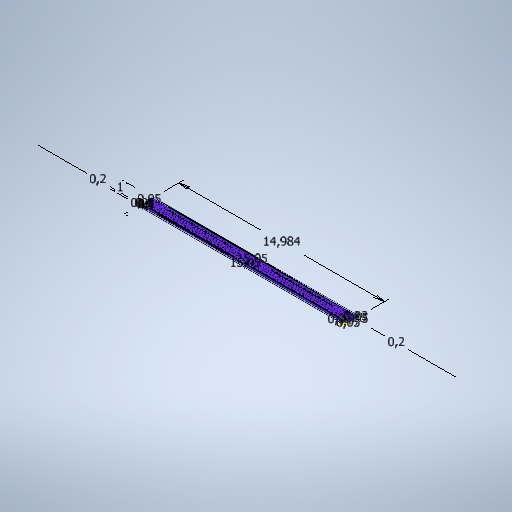
# Autodesk Inventor part: sensor_electrodo
Saved by Autodesk Inventor 2025.2 (Build 292293000, 293)
## iProperties
Created: 2025-03-24
Part Number: sensor_electrodo
Material: Genérico
Document SubType Name: Modeling
Designer: julia
Density: 1 g/cm^3
Appearance: Vidriado - Ladrillo refractario
Author: julia
Autodesk Inventor part; units mm, degrees
ref_plane "YZ Plane" through (0, 0, 0) normal (1, 0, 0) x (0, 1, 0)
ref_plane "XZ Plane" through (0, 0, 0) normal (0, 1, 0) x (-1, 0, 0)
ref_plane "XY Plane" through (0, 0, 0) normal (0, 0, 1) x (1, 0, 0)
sketch "Boceto1" plane through (0, 0, 0) normal (0, 1, 0) x (-1, 0, 0)
  line L0 (0, 0) -> (14.984, 0)
  line L1 (14.984, 0) -> (14.984, -1)
  line L2 (14.984, -1) -> (0, -1)
  line L3 (0, -1) -> (0, 0)
  line L4 (-0.05, -0.23) -> (0, -0.23)
  line L5 (-0.0448, -0.147) -> (-0.0448, -0.3192)
  line L6 (-0.0448, -0.23) -> (15.0052, -0.23)
  line L7 (15.0052, -0.23) -> (15.0052, -0.28)
  line L8 (15.0052, -0.28) -> (14.9052, -0.28)
  line L9 (14.9052, -0.28) -> (14.9052, -0.38)
  line L10 (14.9052, -0.38) -> (14.8052, -0.38)
  line L11 (14.8052, -0.38) -> (14.8052, -0.28)
  line L12 (14.8052, -0.28) -> (14.7052, -0.28)
  line L13 (14.7052, -0.28) -> (14.7052, -0.38)
  line L14 (14.7052, -0.38) -> (14.6052, -0.38)
  line L15 (14.6052, -0.38) -> (14.6052, -0.28)
  line L16 (14.6052, -0.28) -> (14.5052, -0.28)
  line L17 (14.5052, -0.28) -> (14.5052, -0.38)
  line L18 (14.5052, -0.38) -> (14.4052, -0.38)
  line L19 (14.4052, -0.38) -> (14.4052, -0.28)
  line L20 (14.4052, -0.28) -> (14.3052, -0.28)
  line L21 (14.3052, -0.28) -> (14.3052, -0.38)
  line L22 (14.3052, -0.38) -> (14.2052, -0.38)
  line L23 (14.2052, -0.38) -> (14.2052, -0.28)
  line L24 (14.2052, -0.28) -> (14.1052, -0.28)
  line L25 (14.1052, -0.28) -> (14.1052, -0.38)
  line L26 (14.1052, -0.38) -> (14.0052, -0.38)
  line L27 (14.0052, -0.38) -> (14.0052, -0.28)
  line L28 (14.0052, -0.28) -> (13.9052, -0.28)
  line L29 (13.9052, -0.28) -> (13.9052, -0.38)
  line L30 (13.9052, -0.38) -> (13.8052, -0.38)
  line L31 (13.8052, -0.38) -> (13.8052, -0.28)
  line L32 (13.8052, -0.28) -> (13.7052, -0.28)
  line L33 (13.7052, -0.28) -> (13.7052, -0.38)
  line L34 (13.7052, -0.38) -> (13.6052, -0.38)
  line L35 (13.6052, -0.38) -> (13.6052, -0.28)
  line L36 (13.6052, -0.28) -> (13.5052, -0.28)
  line L37 (13.5052, -0.28) -> (13.5052, -0.38)
  line L38 (13.5052, -0.38) -> (13.4052, -0.38)
  line L39 (13.4052, -0.38) -> (13.4052, -0.28)
  line L40 (13.4052, -0.28) -> (13.3052, -0.28)
  line L41 (13.3052, -0.28) -> (13.3052, -0.38)
  line L42 (13.3052, -0.38) -> (13.2052, -0.38)
  line L43 (13.2052, -0.38) -> (13.2052, -0.28)
  line L44 (13.2052, -0.28) -> (13.1052, -0.28)
  line L45 (13.1052, -0.28) -> (13.1052, -0.38)
  line L46 (13.1052, -0.38) -> (13.0052, -0.38)
  line L47 (13.0052, -0.38) -> (13.0052, -0.28)
  line L48 (13.0052, -0.28) -> (12.9052, -0.28)
  line L49 (12.9052, -0.28) -> (12.9052, -0.38)
  line L50 (12.9052, -0.38) -> (12.8052, -0.38)
  line L51 (12.8052, -0.38) -> (12.8052, -0.28)
  line L52 (12.8052, -0.28) -> (12.7052, -0.28)
  line L53 (12.7052, -0.28) -> (12.7052, -0.38)
  line L54 (12.7052, -0.38) -> (12.6052, -0.38)
  line L55 (12.6052, -0.38) -> (12.6052, -0.28)
  line L56 (12.6052, -0.28) -> (12.5052, -0.28)
  line L57 (12.5052, -0.28) -> (12.5052, -0.38)
  line L58 (12.5052, -0.38) -> (12.4052, -0.38)
  line L59 (12.4052, -0.38) -> (12.4052, -0.28)
  line L60 (12.4052, -0.28) -> (12.3052, -0.28)
  line L61 (12.3052, -0.28) -> (12.3052, -0.38)
  line L62 (12.3052, -0.38) -> (12.2052, -0.38)
  line L63 (12.2052, -0.38) -> (12.2052, -0.28)
  line L64 (12.2052, -0.28) -> (12.1052, -0.28)
  line L65 (12.1052, -0.28) -> (12.1052, -0.38)
  line L66 (12.1052, -0.38) -> (12.0052, -0.38)
  line L67 (12.0052, -0.38) -> (12.0052, -0.28)
  line L68 (12.0052, -0.28) -> (11.9052, -0.28)
  line L69 (11.9052, -0.28) -> (11.9052, -0.38)
  line L70 (11.9052, -0.38) -> (11.8052, -0.38)
  line L71 (11.8052, -0.38) -> (11.8052, -0.28)
  line L72 (11.8052, -0.28) -> (11.7052, -0.28)
  line L73 (11.7052, -0.28) -> (11.7052, -0.38)
  line L74 (11.7052, -0.38) -> (11.6052, -0.38)
  line L75 (11.6052, -0.38) -> (11.6052, -0.28)
  line L76 (11.6052, -0.28) -> (11.5052, -0.28)
  line L77 (11.5052, -0.28) -> (11.5052, -0.38)
  line L78 (11.5052, -0.38) -> (11.4052, -0.38)
  line L79 (11.4052, -0.38) -> (11.4052, -0.28)
  line L80 (11.4052, -0.28) -> (11.3052, -0.28)
  line L81 (11.3052, -0.28) -> (11.3052, -0.38)
  line L82 (11.3052, -0.38) -> (11.2052, -0.38)
  line L83 (11.2052, -0.38) -> (11.2052, -0.28)
  line L84 (11.2052, -0.28) -> (11.1052, -0.28)
  line L85 (11.1052, -0.28) -> (11.1052, -0.38)
  line L86 (11.1052, -0.38) -> (11.0052, -0.38)
  line L87 (11.0052, -0.38) -> (11.0052, -0.28)
  line L88 (11.0052, -0.28) -> (10.9052, -0.28)
  line L89 (10.9052, -0.28) -> (10.9052, -0.38)
  line L90 (10.9052, -0.38) -> (10.8052, -0.38)
  line L91 (10.8052, -0.38) -> (10.8052, -0.28)
  line L92 (10.8052, -0.28) -> (10.7052, -0.28)
  line L93 (10.7052, -0.28) -> (10.7052, -0.38)
  line L94 (10.7052, -0.38) -> (10.6052, -0.38)
  line L95 (10.6052, -0.38) -> (10.6052, -0.28)
  line L96 (10.6052, -0.28) -> (10.5052, -0.28)
  line L97 (10.5052, -0.28) -> (10.5052, -0.38)
  line L98 (10.5052, -0.38) -> (10.4052, -0.38)
  line L99 (10.4052, -0.38) -> (10.4052, -0.28)
  line L100 (10.4052, -0.28) -> (10.3052, -0.28)
  line L101 (10.3052, -0.28) -> (10.3052, -0.38)
  line L102 (10.3052, -0.38) -> (10.2052, -0.38)
  line L103 (10.2052, -0.38) -> (10.2052, -0.28)
  line L104 (10.2052, -0.28) -> (10.1052, -0.28)
  line L105 (10.1052, -0.28) -> (10.1052, -0.38)
  line L106 (10.1052, -0.38) -> (10.0052, -0.38)
  line L107 (10.0052, -0.38) -> (10.0052, -0.28)
  line L108 (10.0052, -0.28) -> (9.9052, -0.28)
  line L109 (9.9052, -0.28) -> (9.9052, -0.38)
  line L110 (9.9052, -0.38) -> (9.8052, -0.38)
  line L111 (9.8052, -0.38) -> (9.8052, -0.28)
  line L112 (9.8052, -0.28) -> (9.7052, -0.28)
  line L113 (9.7052, -0.28) -> (9.7052, -0.38)
  line L114 (9.7052, -0.38) -> (9.6052, -0.38)
  line L115 (9.6052, -0.38) -> (9.6052, -0.28)
  line L116 (9.6052, -0.28) -> (9.5052, -0.28)
  line L117 (9.5052, -0.28) -> (9.5052, -0.38)
  line L118 (9.5052, -0.38) -> (9.4052, -0.38)
  line L119 (9.4052, -0.38) -> (9.4052, -0.28)
  line L120 (9.4052, -0.28) -> (9.3052, -0.28)
  line L121 (9.3052, -0.28) -> (9.3052, -0.38)
  line L122 (9.3052, -0.38) -> (9.2052, -0.38)
  line L123 (9.2052, -0.38) -> (9.2052, -0.28)
  line L124 (9.2052, -0.28) -> (9.1052, -0.28)
  line L125 (9.1052, -0.28) -> (9.1052, -0.38)
  line L126 (9.1052, -0.38) -> (9.0052, -0.38)
  line L127 (9.0052, -0.38) -> (9.0052, -0.28)
  line L128 (9.0052, -0.28) -> (8.9052, -0.28)
  line L129 (8.9052, -0.28) -> (8.9052, -0.38)
  line L130 (8.9052, -0.38) -> (8.8052, -0.38)
  line L131 (8.8052, -0.38) -> (8.8052, -0.28)
  line L132 (8.8052, -0.28) -> (8.7052, -0.28)
  line L133 (8.7052, -0.28) -> (8.7052, -0.38)
  line L134 (8.7052, -0.38) -> (8.6052, -0.38)
  line L135 (8.6052, -0.38) -> (8.6052, -0.28)
  line L136 (8.6052, -0.28) -> (8.5052, -0.28)
  line L137 (8.5052, -0.28) -> (8.5052, -0.38)
  line L138 (8.5052, -0.38) -> (8.4052, -0.38)
  line L139 (8.4052, -0.38) -> (8.4052, -0.28)
  line L140 (8.4052, -0.28) -> (8.3052, -0.28)
  line L141 (8.3052, -0.28) -> (8.3052, -0.38)
  line L142 (8.3052, -0.38) -> (8.2052, -0.38)
  line L143 (8.2052, -0.38) -> (8.2052, -0.28)
  line L144 (8.2052, -0.28) -> (8.1052, -0.28)
  line L145 (8.1052, -0.28) -> (8.1052, -0.38)
  line L146 (8.1052, -0.38) -> (8.0052, -0.38)
  line L147 (8.0052, -0.38) -> (8.0052, -0.28)
  line L148 (8.0052, -0.28) -> (7.9052, -0.28)
  line L149 (7.9052, -0.28) -> (7.9052, -0.38)
  line L150 (7.9052, -0.38) -> (7.8052, -0.38)
  line L151 (7.8052, -0.38) -> (7.8052, -0.28)
  line L152 (7.8052, -0.28) -> (7.7052, -0.28)
  line L153 (7.7052, -0.28) -> (7.7052, -0.38)
  line L154 (7.7052, -0.38) -> (7.6052, -0.38)
  line L155 (7.6052, -0.38) -> (7.6052, -0.28)
  line L156 (7.6052, -0.28) -> (7.5052, -0.28)
  line L157 (7.5052, -0.28) -> (7.5052, -0.38)
  line L158 (7.5052, -0.38) -> (7.4052, -0.38)
  line L159 (7.4052, -0.38) -> (7.4052, -0.28)
  line L160 (7.4052, -0.28) -> (7.3052, -0.28)
  line L161 (7.3052, -0.28) -> (7.3052, -0.38)
  line L162 (7.3052, -0.38) -> (7.2052, -0.38)
  line L163 (7.2052, -0.38) -> (7.2052, -0.28)
  line L164 (7.2052, -0.28) -> (7.1052, -0.28)
  line L165 (7.1052, -0.28) -> (7.1052, -0.38)
  line L166 (7.1052, -0.38) -> (7.0052, -0.38)
  line L167 (7.0052, -0.38) -> (7.0052, -0.28)
  line L168 (7.0052, -0.28) -> (6.9052, -0.28)
  line L169 (6.9052, -0.28) -> (6.9052, -0.38)
  line L170 (6.9052, -0.38) -> (6.8052, -0.38)
  line L171 (6.8052, -0.38) -> (6.8052, -0.28)
  line L172 (6.8052, -0.28) -> (6.7052, -0.28)
  line L173 (6.7052, -0.28) -> (6.7052, -0.38)
  line L174 (6.7052, -0.38) -> (6.6052, -0.38)
  line L175 (6.6052, -0.38) -> (6.6052, -0.28)
  line L176 (6.6052, -0.28) -> (6.5052, -0.28)
  line L177 (6.5052, -0.28) -> (6.5052, -0.38)
  line L178 (6.5052, -0.38) -> (6.4052, -0.38)
  line L179 (6.4052, -0.38) -> (6.4052, -0.28)
  line L180 (6.4052, -0.28) -> (6.3052, -0.28)
  line L181 (6.3052, -0.28) -> (6.3052, -0.38)
  line L182 (6.3052, -0.38) -> (6.2052, -0.38)
  line L183 (6.2052, -0.38) -> (6.2052, -0.28)
  line L184 (6.2052, -0.28) -> (6.1052, -0.28)
  line L185 (6.1052, -0.28) -> (6.1052, -0.38)
  line L186 (6.1052, -0.38) -> (6.0052, -0.38)
  line L187 (6.0052, -0.38) -> (6.0052, -0.28)
  line L188 (6.0052, -0.28) -> (5.9052, -0.28)
  line L189 (5.9052, -0.28) -> (5.9052, -0.38)
  line L190 (5.9052, -0.38) -> (5.8052, -0.38)
  line L191 (5.8052, -0.38) -> (5.8052, -0.28)
  line L192 (5.8052, -0.28) -> (5.7052, -0.28)
  line L193 (5.7052, -0.28) -> (5.7052, -0.38)
  line L194 (5.7052, -0.38) -> (5.6052, -0.38)
  line L195 (5.6052, -0.38) -> (5.6052, -0.28)
  line L196 (5.6052, -0.28) -> (5.5052, -0.28)
  line L197 (5.5052, -0.28) -> (5.5052, -0.38)
  line L198 (5.5052, -0.38) -> (5.4052, -0.38)
  line L199 (5.4052, -0.38) -> (5.4052, -0.28)
  line L200 (5.4052, -0.28) -> (5.3052, -0.28)
  line L201 (5.3052, -0.28) -> (5.3052, -0.38)
  line L202 (5.3052, -0.38) -> (5.2052, -0.38)
  line L203 (5.2052, -0.38) -> (5.2052, -0.28)
  line L204 (5.2052, -0.28) -> (5.1052, -0.28)
  line L205 (5.1052, -0.28) -> (5.1052, -0.38)
  line L206 (5.1052, -0.38) -> (5.0052, -0.38)
  line L207 (5.0052, -0.38) -> (5.0052, -0.28)
  line L208 (5.0052, -0.28) -> (4.9052, -0.28)
  line L209 (4.9052, -0.28) -> (4.9052, -0.38)
  line L210 (4.9052, -0.38) -> (4.8052, -0.38)
  line L211 (4.8052, -0.38) -> (4.8052, -0.28)
  line L212 (4.8052, -0.28) -> (4.7052, -0.28)
  line L213 (4.7052, -0.28) -> (4.7052, -0.38)
  line L214 (4.7052, -0.38) -> (4.6052, -0.38)
  line L215 (4.6052, -0.38) -> (4.6052, -0.28)
  line L216 (4.6052, -0.28) -> (4.5052, -0.28)
  line L217 (4.5052, -0.28) -> (4.5052, -0.38)
  line L218 (4.5052, -0.38) -> (4.4052, -0.38)
  line L219 (4.4052, -0.38) -> (4.4052, -0.28)
  line L220 (4.4052, -0.28) -> (4.3052, -0.28)
  line L221 (4.3052, -0.28) -> (4.3052, -0.38)
  line L222 (4.3052, -0.38) -> (4.2052, -0.38)
  line L223 (4.2052, -0.38) -> (4.2052, -0.28)
  line L224 (4.2052, -0.28) -> (4.1052, -0.28)
  line L225 (4.1052, -0.28) -> (4.1052, -0.38)
  line L226 (4.1052, -0.38) -> (4.0052, -0.38)
  line L227 (4.0052, -0.38) -> (4.0052, -0.28)
  line L228 (4.0052, -0.28) -> (3.9052, -0.28)
  line L229 (3.9052, -0.28) -> (3.9052, -0.38)
  line L230 (3.9052, -0.38) -> (3.8052, -0.38)
  line L231 (3.8052, -0.38) -> (3.8052, -0.28)
  line L232 (3.8052, -0.28) -> (3.7052, -0.28)
  line L233 (3.7052, -0.28) -> (3.7052, -0.38)
  line L234 (3.7052, -0.38) -> (3.6052, -0.38)
  line L235 (3.6052, -0.38) -> (3.6052, -0.28)
  line L236 (3.6052, -0.28) -> (3.5052, -0.28)
  line L237 (3.5052, -0.28) -> (3.5052, -0.38)
  line L238 (3.5052, -0.38) -> (3.4052, -0.38)
  line L239 (3.4052, -0.38) -> (3.4052, -0.28)
  line L240 (3.4052, -0.28) -> (3.3052, -0.28)
  line L241 (3.3052, -0.28) -> (3.3052, -0.38)
  line L242 (3.3052, -0.38) -> (3.2052, -0.38)
  line L243 (3.2052, -0.38) -> (3.2052, -0.28)
  line L244 (3.2052, -0.28) -> (3.1052, -0.28)
  line L245 (3.1052, -0.28) -> (3.1052, -0.38)
  line L246 (3.1052, -0.38) -> (3.0052, -0.38)
  line L247 (3.0052, -0.38) -> (3.0052, -0.28)
  line L248 (3.0052, -0.28) -> (2.9052, -0.28)
  line L249 (2.9052, -0.28) -> (2.9052, -0.38)
  line L250 (2.9052, -0.38) -> (2.8052, -0.38)
  line L251 (2.8052, -0.38) -> (2.8052, -0.28)
  line L252 (2.8052, -0.28) -> (2.7052, -0.28)
  line L253 (2.7052, -0.28) -> (2.7052, -0.38)
  line L254 (2.7052, -0.38) -> (2.6052, -0.38)
  line L255 (2.6052, -0.38) -> (2.6052, -0.28)
  line L256 (2.6052, -0.28) -> (2.5052, -0.28)
  line L257 (2.5052, -0.28) -> (2.5052, -0.38)
  line L258 (2.5052, -0.38) -> (2.4052, -0.38)
  line L259 (2.4052, -0.38) -> (2.4052, -0.28)
  line L260 (2.4052, -0.28) -> (2.3052, -0.28)
  line L261 (2.3052, -0.28) -> (2.3052, -0.38)
  line L262 (2.3052, -0.38) -> (2.2052, -0.38)
  line L263 (2.2052, -0.38) -> (2.2052, -0.28)
  line L264 (2.2052, -0.28) -> (2.1052, -0.28)
  line L265 (2.1052, -0.28) -> (2.1052, -0.38)
  line L266 (2.1052, -0.38) -> (2.0052, -0.38)
  line L267 (2.0052, -0.38) -> (2.0052, -0.28)
  line L268 (2.0052, -0.28) -> (1.9052, -0.28)
  line L269 (1.9052, -0.28) -> (1.9052, -0.38)
  line L270 (1.9052, -0.38) -> (1.8052, -0.38)
  line L271 (1.8052, -0.38) -> (1.8052, -0.28)
  line L272 (1.8052, -0.28) -> (1.7052, -0.28)
  line L273 (1.7052, -0.28) -> (1.7052, -0.38)
  line L274 (1.7052, -0.38) -> (1.6052, -0.38)
  line L275 (1.6052, -0.38) -> (1.6052, -0.28)
  line L276 (1.6052, -0.28) -> (1.5052, -0.28)
  line L277 (1.5052, -0.28) -> (1.5052, -0.38)
  line L278 (1.5052, -0.38) -> (1.4052, -0.38)
  line L279 (1.4052, -0.38) -> (1.4052, -0.28)
  line L280 (1.4052, -0.28) -> (1.3052, -0.28)
  line L281 (1.3052, -0.28) -> (1.3052, -0.38)
  line L282 (1.3052, -0.38) -> (1.2052, -0.38)
  line L283 (1.2052, -0.38) -> (1.2052, -0.28)
  line L284 (1.2052, -0.28) -> (1.1052, -0.28)
  line L285 (1.1052, -0.28) -> (1.1052, -0.38)
  line L286 (1.1052, -0.38) -> (1.0052, -0.38)
  line L287 (1.0052, -0.38) -> (1.0052, -0.28)
  line L288 (1.0052, -0.28) -> (0.9052, -0.28)
  line L289 (0.9052, -0.28) -> (0.9052, -0.38)
  line L290 (0.9052, -0.38) -> (0.8052, -0.38)
  line L291 (0.8052, -0.38) -> (0.8052, -0.28)
  line L292 (0.8052, -0.28) -> (0.7052, -0.28)
  line L293 (0.7052, -0.28) -> (0.7052, -0.38)
  line L294 (0.7052, -0.38) -> (0.6052, -0.38)
  line L295 (0.6052, -0.38) -> (0.6052, -0.28)
  line L296 (0.6052, -0.28) -> (0.5052, -0.28)
  line L297 (0.5052, -0.28) -> (0.5052, -0.38)
  line L298 (0.5052, -0.38) -> (0.4052, -0.38)
  line L299 (0.4052, -0.38) -> (0.4052, -0.28)
  line L300 (0.4052, -0.28) -> (0.3052, -0.28)
  line L301 (0.3052, -0.28) -> (0.3052, -0.38)
  line L302 (0.3052, -0.38) -> (0.2052, -0.38)
  line L303 (0.2052, -0.38) -> (0.2052, -0.28)
  line L304 (0.2052, -0.28) -> (-0.0448, -0.28)
  line L305 (-0.0448, -0.28) -> (-0.0448, -1.0485)
  line L306 (-0.0448, -0.77) -> (15.0052, -0.77)
  line L307 (-0.0448, -0.77) -> (-0.0448, -0.72)
  line L308 (-0.0448, -0.72) -> (0.1052, -0.72)
  line L309 (0.1052, -0.72) -> (0.1052, -0.62)
  line L310 (0.1052, -0.62) -> (0.2052, -0.62)
  line L311 (0.2052, -0.62) -> (0.2052, -0.72)
  line L312 (15.0052, -0.77) -> (15.0052, -0.72)
  line L313 (0.2052, -0.72) -> (0.3052, -0.72)
  line L314 (0.3052, -0.72) -> (0.3052, -0.62)
  line L315 (0.3052, -0.62) -> (0.4052, -0.62)
  line L316 (0.4052, -0.62) -> (0.4052, -0.72)
  line L317 (0.4052, -0.72) -> (0.5052, -0.72)
  line L318 (0.5052, -0.72) -> (0.5052, -0.62)
  line L319 (0.5052, -0.62) -> (0.6052, -0.62)
  line L320 (0.6052, -0.62) -> (0.6052, -0.72)
  line L321 (0.6052, -0.72) -> (0.7052, -0.72)
  line L322 (0.7052, -0.72) -> (0.7052, -0.62)
  line L323 (0.7052, -0.62) -> (0.8052, -0.62)
  line L324 (0.8052, -0.62) -> (0.8052, -0.72)
  line L325 (0.8052, -0.72) -> (0.9052, -0.72)
  line L326 (0.9052, -0.72) -> (0.9052, -0.62)
  line L327 (0.9052, -0.62) -> (1.0052, -0.62)
  line L328 (1.0052, -0.62) -> (1.0052, -0.72)
  line L329 (1.0052, -0.72) -> (1.1052, -0.72)
  line L330 (1.1052, -0.72) -> (1.1052, -0.62)
  line L331 (1.1052, -0.62) -> (1.2052, -0.62)
  line L332 (1.2052, -0.62) -> (1.2052, -0.72)
  line L333 (1.2052, -0.72) -> (1.3052, -0.72)
  line L334 (1.3052, -0.72) -> (1.3052, -0.62)
  line L335 (1.3052, -0.62) -> (1.4052, -0.62)
  line L336 (1.4052, -0.62) -> (1.4052, -0.72)
  line L337 (1.4052, -0.72) -> (1.5052, -0.72)
  line L338 (1.5052, -0.72) -> (1.5052, -0.62)
  line L339 (1.5052, -0.62) -> (1.6052, -0.62)
  line L340 (1.6052, -0.62) -> (1.6052, -0.72)
  line L341 (1.6052, -0.72) -> (1.7052, -0.72)
  line L342 (1.7052, -0.72) -> (1.7052, -0.62)
  line L343 (1.7052, -0.62) -> (1.8052, -0.62)
  line L344 (1.8052, -0.62) -> (1.8052, -0.72)
  line L345 (1.8052, -0.72) -> (1.9052, -0.72)
  line L346 (1.9052, -0.72) -> (1.9052, -0.62)
  line L347 (1.9052, -0.62) -> (2.0052, -0.62)
  line L348 (2.0052, -0.62) -> (2.0052, -0.72)
  line L349 (2.0052, -0.72) -> (2.1052, -0.72)
  line L350 (2.1052, -0.72) -> (2.1052, -0.62)
  line L351 (2.1052, -0.62) -> (2.2052, -0.62)
  line L352 (2.2052, -0.62) -> (2.2052, -0.72)
  line L353 (2.2052, -0.72) -> (2.3052, -0.72)
  line L354 (2.3052, -0.72) -> (2.3052, -0.62)
  line L355 (2.3052, -0.62) -> (2.4052, -0.62)
  line L356 (2.4052, -0.62) -> (2.4052, -0.72)
  line L357 (2.4052, -0.72) -> (2.5052, -0.72)
  line L358 (2.5052, -0.72) -> (2.5052, -0.62)
  line L359 (2.5052, -0.62) -> (2.6052, -0.62)
  line L360 (2.6052, -0.62) -> (2.6052, -0.72)
  line L361 (2.6052, -0.72) -> (2.7052, -0.72)
  line L362 (2.7052, -0.72) -> (2.7052, -0.62)
  line L363 (2.7052, -0.62) -> (2.8052, -0.62)
  line L364 (2.8052, -0.62) -> (2.8052, -0.72)
  line L365 (2.8052, -0.72) -> (2.9052, -0.72)
  line L366 (2.9052, -0.72) -> (2.9052, -0.62)
  line L367 (2.9052, -0.62) -> (3.0052, -0.62)
  line L368 (3.0052, -0.62) -> (3.0052, -0.72)
  line L369 (3.0052, -0.72) -> (3.1052, -0.72)
  line L370 (3.1052, -0.72) -> (3.1052, -0.62)
  line L371 (3.1052, -0.62) -> (3.2052, -0.62)
  line L372 (3.2052, -0.62) -> (3.2052, -0.72)
  line L373 (3.2052, -0.72) -> (3.3052, -0.72)
  line L374 (3.3052, -0.72) -> (3.3052, -0.62)
  line L375 (3.3052, -0.62) -> (3.4052, -0.62)
  line L376 (3.4052, -0.62) -> (3.4052, -0.72)
  line L377 (3.4052, -0.72) -> (3.5052, -0.72)
  line L378 (3.5052, -0.72) -> (3.5052, -0.62)
  line L379 (3.5052, -0.62) -> (3.6052, -0.62)
  line L380 (3.6052, -0.62) -> (3.6052, -0.72)
  line L381 (3.6052, -0.72) -> (3.7052, -0.72)
  line L382 (3.7052, -0.72) -> (3.7052, -0.62)
  line L383 (3.7052, -0.62) -> (3.8052, -0.62)
  line L384 (3.8052, -0.62) -> (3.8052, -0.72)
  line L385 (3.8052, -0.72) -> (3.9052, -0.72)
  line L386 (3.9052, -0.72) -> (3.9052, -0.62)
  line L387 (3.9052, -0.62) -> (4.0052, -0.62)
  line L388 (4.0052, -0.62) -> (4.0052, -0.72)
  line L389 (4.0052, -0.72) -> (4.1052, -0.72)
  line L390 (4.1052, -0.72) -> (4.1052, -0.62)
  line L391 (4.1052, -0.62) -> (4.2052, -0.62)
  line L392 (4.2052, -0.62) -> (4.2052, -0.72)
  line L393 (4.2052, -0.72) -> (4.3052, -0.72)
  line L394 (4.3052, -0.72) -> (4.3052, -0.62)
  line L395 (4.3052, -0.62) -> (4.4052, -0.62)
  line L396 (4.4052, -0.62) -> (4.4052, -0.72)
  line L397 (4.4052, -0.72) -> (4.5052, -0.72)
  line L398 (4.5052, -0.72) -> (4.5052, -0.62)
  line L399 (4.5052, -0.62) -> (4.6052, -0.62)
  line L400 (4.6052, -0.62) -> (4.6052, -0.72)
  line L401 (4.6052, -0.72) -> (4.7052, -0.72)
  line L402 (4.7052, -0.72) -> (4.7052, -0.62)
  line L403 (4.7052, -0.62) -> (4.8052, -0.62)
  line L404 (4.8052, -0.62) -> (4.8052, -0.72)
  line L405 (4.8052, -0.72) -> (4.9052, -0.72)
  line L406 (4.9052, -0.72) -> (4.9052, -0.62)
  line L407 (4.9052, -0.62) -> (5.0052, -0.62)
  line L408 (5.0052, -0.62) -> (5.0052, -0.72)
  line L409 (5.0052, -0.72) -> (5.1052, -0.72)
  line L410 (5.1052, -0.72) -> (5.1052, -0.62)
  line L411 (5.1052, -0.62) -> (5.2052, -0.62)
  line L412 (5.2052, -0.62) -> (5.2052, -0.72)
  line L413 (5.2052, -0.72) -> (5.3052, -0.72)
  line L414 (5.3052, -0.72) -> (5.3052, -0.62)
  line L415 (5.3052, -0.62) -> (5.4052, -0.62)
  line L416 (5.4052, -0.62) -> (5.4052, -0.72)
  line L417 (5.4052, -0.72) -> (5.5052, -0.72)
  line L418 (5.5052, -0.72) -> (5.5052, -0.62)
  line L419 (5.5052, -0.62) -> (5.6052, -0.62)
  line L420 (5.6052, -0.62) -> (5.6052, -0.72)
  line L421 (5.6052, -0.72) -> (5.7052, -0.72)
  line L422 (5.7052, -0.72) -> (5.7052, -0.62)
  line L423 (5.7052, -0.62) -> (5.8052, -0.62)
  line L424 (5.8052, -0.62) -> (5.8052, -0.72)
  line L425 (5.8052, -0.72) -> (5.9052, -0.72)
  line L426 (5.9052, -0.72) -> (5.9052, -0.62)
  line L427 (5.9052, -0.62) -> (6.0052, -0.62)
  line L428 (6.0052, -0.62) -> (6.0052, -0.72)
  line L429 (6.0052, -0.72) -> (6.1052, -0.72)
  line L430 (6.1052, -0.72) -> (6.1052, -0.62)
  line L431 (6.1052, -0.62) -> (6.2052, -0.62)
  line L432 (6.2052, -0.62) -> (6.2052, -0.72)
  line L433 (6.2052, -0.72) -> (6.3052, -0.72)
  line L434 (6.3052, -0.72) -> (6.3052, -0.62)
  line L435 (6.3052, -0.62) -> (6.4052, -0.62)
  line L436 (6.4052, -0.62) -> (6.4052, -0.72)
  line L437 (6.4052, -0.72) -> (6.5052, -0.72)
  line L438 (6.5052, -0.72) -> (6.5052, -0.62)
  line L439 (6.5052, -0.62) -> (6.6052, -0.62)
  line L440 (6.6052, -0.62) -> (6.6052, -0.72)
  line L441 (6.6052, -0.72) -> (6.7052, -0.72)
  line L442 (6.7052, -0.72) -> (6.7052, -0.62)
  line L443 (6.7052, -0.62) -> (6.8052, -0.62)
  line L444 (6.8052, -0.62) -> (6.8052, -0.72)
  line L445 (6.8052, -0.72) -> (6.9052, -0.72)
  line L446 (6.9052, -0.72) -> (6.9052, -0.62)
  line L447 (6.9052, -0.62) -> (7.0052, -0.62)
  line L448 (7.0052, -0.62) -> (7.0052, -0.72)
  line L449 (7.0052, -0.72) -> (7.1052, -0.72)
  line L450 (7.1052, -0.72) -> (7.1052, -0.62)
  line L451 (7.1052, -0.62) -> (7.2052, -0.62)
  line L452 (7.2052, -0.62) -> (7.2052, -0.72)
  line L453 (7.2052, -0.72) -> (7.3052, -0.72)
  line L454 (7.3052, -0.72) -> (7.3052, -0.62)
  line L455 (7.3052, -0.62) -> (7.4052, -0.62)
  line L456 (7.4052, -0.62) -> (7.4052, -0.72)
  line L457 (7.4052, -0.72) -> (7.5052, -0.72)
  line L458 (7.5052, -0.72) -> (7.5052, -0.62)
  line L459 (7.5052, -0.62) -> (7.6052, -0.62)
  line L460 (7.6052, -0.62) -> (7.6052, -0.72)
  line L461 (7.6052, -0.72) -> (7.7052, -0.72)
  line L462 (7.7052, -0.72) -> (7.7052, -0.62)
  line L463 (7.7052, -0.62) -> (7.8052, -0.62)
  line L464 (7.8052, -0.62) -> (7.8052, -0.72)
  line L465 (7.8052, -0.72) -> (7.9052, -0.72)
  line L466 (7.9052, -0.72) -> (7.9052, -0.62)
  line L467 (7.9052, -0.62) -> (8.0052, -0.62)
  line L468 (8.0052, -0.62) -> (8.0052, -0.72)
  line L469 (8.0052, -0.72) -> (8.1052, -0.72)
  line L470 (8.1052, -0.72) -> (8.1052, -0.62)
  line L471 (8.1052, -0.62) -> (8.2052, -0.62)
  line L472 (8.2052, -0.62) -> (8.2052, -0.72)
  line L473 (8.2052, -0.72) -> (8.3052, -0.72)
  line L474 (8.3052, -0.72) -> (8.3052, -0.62)
  line L475 (8.3052, -0.62) -> (8.4052, -0.62)
  line L476 (8.4052, -0.62) -> (8.4052, -0.72)
  line L477 (8.4052, -0.72) -> (8.5052, -0.72)
  line L478 (8.5052, -0.72) -> (8.5052, -0.62)
  line L479 (8.5052, -0.62) -> (8.6052, -0.62)
  line L480 (8.6052, -0.62) -> (8.6052, -0.72)
  line L481 (8.6052, -0.72) -> (8.7052, -0.72)
  line L482 (8.7052, -0.72) -> (8.7052, -0.62)
  line L483 (8.7052, -0.62) -> (8.8052, -0.62)
  line L484 (8.8052, -0.62) -> (8.8052, -0.72)
  line L485 (8.8052, -0.72) -> (8.9052, -0.72)
  line L486 (8.9052, -0.72) -> (8.9052, -0.62)
  line L487 (8.9052, -0.62) -> (9.0052, -0.62)
  line L488 (9.0052, -0.62) -> (9.0052, -0.72)
  line L489 (9.0052, -0.72) -> (9.1052, -0.72)
  line L490 (9.1052, -0.72) -> (9.1052, -0.62)
  line L491 (9.1052, -0.62) -> (9.2052, -0.62)
  line L492 (9.2052, -0.62) -> (9.2052, -0.72)
  line L493 (9.2052, -0.72) -> (9.3052, -0.72)
  line L494 (9.3052, -0.72) -> (9.3052, -0.62)
  line L495 (9.3052, -0.62) -> (9.4052, -0.62)
  line L496 (9.4052, -0.62) -> (9.4052, -0.72)
  line L497 (9.4052, -0.72) -> (9.5052, -0.72)
  line L498 (9.5052, -0.72) -> (9.5052, -0.62)
  line L499 (9.5052, -0.62) -> (9.6052, -0.62)
  line L500 (9.6052, -0.62) -> (9.6052, -0.72)
  line L501 (9.6052, -0.72) -> (9.7052, -0.72)
  line L502 (9.7052, -0.72) -> (9.7052, -0.62)
  line L503 (9.7052, -0.62) -> (9.8052, -0.62)
  line L504 (9.8052, -0.62) -> (9.8052, -0.72)
  line L505 (9.8052, -0.72) -> (9.9052, -0.72)
  line L506 (9.9052, -0.72) -> (9.9052, -0.62)
  line L507 (9.9052, -0.62) -> (10.0052, -0.62)
  line L508 (10.0052, -0.62) -> (10.0052, -0.72)
  line L509 (10.0052, -0.72) -> (10.1052, -0.72)
  line L510 (10.1052, -0.72) -> (10.1052, -0.62)
  line L511 (10.1052, -0.62) -> (10.2052, -0.62)
  line L512 (10.2052, -0.62) -> (10.2052, -0.72)
  line L513 (10.2052, -0.72) -> (10.3052, -0.72)
  line L514 (10.3052, -0.72) -> (10.3052, -0.62)
  line L515 (10.3052, -0.62) -> (10.4052, -0.62)
  line L516 (10.4052, -0.62) -> (10.4052, -0.72)
  line L517 (10.4052, -0.72) -> (10.5052, -0.72)
  line L518 (10.5052, -0.72) -> (10.5052, -0.62)
  line L519 (10.5052, -0.62) -> (10.6052, -0.62)
  line L520 (10.6052, -0.62) -> (10.6052, -0.72)
  line L521 (10.6052, -0.72) -> (10.7052, -0.72)
  line L522 (10.7052, -0.72) -> (10.7052, -0.62)
  line L523 (10.7052, -0.62) -> (10.8052, -0.62)
  line L524 (10.8052, -0.62) -> (10.8052, -0.72)
  line L525 (10.8052, -0.72) -> (10.9052, -0.72)
  line L526 (10.9052, -0.72) -> (10.9052, -0.62)
  line L527 (10.9052, -0.62) -> (11.0052, -0.62)
  line L528 (11.0052, -0.62) -> (11.0052, -0.72)
  line L529 (11.0052, -0.72) -> (11.1052, -0.72)
  line L530 (11.1052, -0.72) -> (11.1052, -0.62)
  line L531 (11.1052, -0.62) -> (11.2052, -0.62)
  line L532 (11.2052, -0.62) -> (11.2052, -0.72)
  line L533 (11.2052, -0.72) -> (11.3052, -0.72)
  line L534 (11.3052, -0.72) -> (11.3052, -0.62)
  line L535 (11.3052, -0.62) -> (11.4052, -0.62)
  line L536 (11.4052, -0.62) -> (11.4052, -0.72)
  line L537 (11.4052, -0.72) -> (11.5052, -0.72)
  line L538 (11.5052, -0.72) -> (11.5052, -0.62)
  line L539 (11.5052, -0.62) -> (11.6052, -0.62)
  line L540 (11.6052, -0.62) -> (11.6052, -0.72)
  line L541 (11.6052, -0.72) -> (11.7052, -0.72)
  line L542 (11.7052, -0.72) -> (11.7052, -0.62)
  line L543 (11.7052, -0.62) -> (11.8052, -0.62)
  line L544 (11.8052, -0.62) -> (11.8052, -0.72)
  line L545 (11.8052, -0.72) -> (11.9052, -0.72)
  line L546 (11.9052, -0.72) -> (11.9052, -0.62)
  line L547 (11.9052, -0.62) -> (12.0052, -0.62)
  line L548 (12.0052, -0.62) -> (12.0052, -0.72)
  line L549 (12.0052, -0.72) -> (12.1052, -0.72)
  line L550 (12.1052, -0.72) -> (12.1052, -0.62)
  line L551 (12.1052, -0.62) -> (12.2052, -0.62)
  line L552 (12.2052, -0.62) -> (12.2052, -0.72)
  line L553 (12.2052, -0.72) -> (12.3052, -0.72)
  line L554 (12.3052, -0.72) -> (12.3052, -0.62)
  line L555 (12.3052, -0.62) -> (12.4052, -0.62)
  line L556 (12.4052, -0.62) -> (12.4052, -0.72)
  line L557 (12.4052, -0.72) -> (12.5052, -0.72)
  line L558 (12.5052, -0.72) -> (12.5052, -0.62)
  line L559 (12.5052, -0.62) -> (12.6052, -0.62)
  line L560 (12.6052, -0.62) -> (12.6052, -0.72)
  line L561 (12.6052, -0.72) -> (12.7052, -0.72)
  line L562 (12.7052, -0.72) -> (12.7052, -0.62)
  line L563 (12.7052, -0.62) -> (12.8052, -0.62)
  line L564 (12.8052, -0.62) -> (12.8052, -0.72)
  line L565 (12.8052, -0.72) -> (12.9052, -0.72)
  line L566 (12.9052, -0.72) -> (12.9052, -0.62)
  line L567 (12.9052, -0.62) -> (13.0052, -0.62)
  line L568 (13.0052, -0.62) -> (13.0052, -0.72)
  line L569 (13.0052, -0.72) -> (13.1052, -0.72)
  line L570 (13.1052, -0.72) -> (13.1052, -0.62)
  line L571 (13.1052, -0.62) -> (13.2052, -0.62)
  line L572 (13.2052, -0.62) -> (13.2052, -0.72)
  line L573 (13.2052, -0.72) -> (13.3052, -0.72)
  line L574 (13.3052, -0.72) -> (13.3052, -0.62)
  line L575 (13.3052, -0.62) -> (13.4052, -0.62)
  line L576 (13.4052, -0.62) -> (13.4052, -0.72)
  line L577 (13.4052, -0.72) -> (13.5052, -0.72)
  line L578 (13.5052, -0.72) -> (13.5052, -0.62)
  line L579 (13.5052, -0.62) -> (13.6052, -0.62)
  line L580 (13.6052, -0.62) -> (13.6052, -0.72)
  line L581 (13.6052, -0.72) -> (13.7052, -0.72)
  line L582 (13.7052, -0.72) -> (13.7052, -0.62)
  line L583 (13.7052, -0.62) -> (13.8052, -0.62)
  line L584 (13.8052, -0.62) -> (13.8052, -0.72)
  line L585 (13.8052, -0.72) -> (13.9052, -0.72)
  line L586 (13.9052, -0.72) -> (13.9052, -0.62)
  line L587 (13.9052, -0.62) -> (14.0052, -0.62)
  line L588 (14.0052, -0.62) -> (14.0052, -0.72)
  line L589 (14.0052, -0.72) -> (14.1052, -0.72)
  line L590 (14.1052, -0.72) -> (14.1052, -0.62)
  line L591 (14.1052, -0.62) -> (14.2052, -0.62)
  line L592 (14.2052, -0.62) -> (14.2052, -0.72)
  line L593 (14.2052, -0.72) -> (14.3052, -0.72)
  line L594 (14.3052, -0.72) -> (14.3052, -0.62)
  line L595 (14.3052, -0.62) -> (14.4052, -0.62)
  line L596 (14.4052, -0.62) -> (14.4052, -0.72)
  line L597 (14.4052, -0.72) -> (14.5052, -0.72)
  line L598 (14.5052, -0.72) -> (14.5052, -0.62)
  line L599 (14.5052, -0.62) -> (14.6052, -0.62)
  line L600 (14.6052, -0.62) -> (14.6052, -0.72)
  line L601 (14.6052, -0.72) -> (14.7052, -0.72)
  line L602 (14.7052, -0.72) -> (14.7052, -0.62)
  line L603 (14.7052, -0.62) -> (14.8052, -0.62)
  line L604 (14.8052, -0.62) -> (14.8052, -0.72)
  line L605 (14.8052, -0.72) -> (14.9052, -0.72)
  line L606 (14.9052, -0.72) -> (15.0052, -0.72)
  point P0 (0.2052, -0.67)
  point P1 (0.4052, -0.67)
  point P2 (0.6052, -0.67)
  point P3 (0.8052, -0.67)
  point P4 (1.0052, -0.67)
  point P5 (1.2052, -0.67)
  point P6 (1.4052, -0.67)
  point P7 (1.6052, -0.67)
  point P8 (1.8052, -0.67)
  point P9 (2.0052, -0.67)
  point P10 (2.2052, -0.67)
  point P11 (2.4052, -0.67)
  point P12 (2.6052, -0.67)
  point P13 (2.8052, -0.67)
  point P14 (3.0052, -0.67)
  point P15 (3.2052, -0.67)
  point P16 (3.4052, -0.67)
  point P17 (3.6052, -0.67)
  point P18 (3.8052, -0.67)
  point P19 (4.0052, -0.67)
  point P20 (4.2052, -0.67)
  point P21 (4.4052, -0.67)
  point P22 (4.6052, -0.67)
  point P23 (4.8052, -0.67)
  point P24 (5.0052, -0.67)
  point P25 (5.2052, -0.67)
  point P26 (5.4052, -0.67)
  point P27 (5.6052, -0.67)
  point P28 (5.8052, -0.67)
  point P29 (6.0052, -0.67)
  point P30 (6.2052, -0.67)
  point P31 (6.4052, -0.67)
  point P32 (6.6052, -0.67)
  point P33 (6.8052, -0.67)
  point P34 (7.0052, -0.67)
  point P35 (7.2052, -0.67)
  point P36 (7.4052, -0.67)
  point P37 (7.6052, -0.67)
  point P38 (7.8052, -0.67)
  point P39 (8.0052, -0.67)
  point P40 (8.2052, -0.67)
  point P41 (8.4052, -0.67)
  point P42 (8.6052, -0.67)
  point P43 (8.8052, -0.67)
  point P44 (9.0052, -0.67)
  point P45 (9.2052, -0.67)
  point P46 (9.4052, -0.67)
  point P47 (9.6052, -0.67)
  point P48 (9.8052, -0.67)
  point P49 (10.0052, -0.67)
  point P50 (10.2052, -0.67)
  point P51 (10.4052, -0.67)
  point P52 (10.6052, -0.67)
  point P53 (10.8052, -0.67)
  point P54 (11.0052, -0.67)
  point P55 (11.2052, -0.67)
  point P56 (11.4052, -0.67)
  point P57 (11.6052, -0.67)
  point P58 (11.8052, -0.67)
  point P59 (12.0052, -0.67)
  point P60 (12.2052, -0.67)
  point P61 (12.4052, -0.67)
  point P62 (12.6052, -0.67)
  point P63 (12.8052, -0.67)
  point P64 (13.0052, -0.67)
  point P65 (13.2052, -0.67)
  point P66 (13.4052, -0.67)
  point P67 (13.6052, -0.67)
  point P68 (13.8052, -0.67)
  point P69 (14.0052, -0.67)
  point P70 (14.2052, -0.67)
  point P71 (14.4052, -0.67)
  point P72 (14.6052, -0.67)
  point P73 (14.8052, -0.67)
  point P74 (0, -0.72)
  point P75 (0, -0.77)
  point P76 (14.984, -0.77)
  point P77 (14.984, -0.72)
  point P78 (14.984, -0.28)
  point P79 (14.984, -0.23)
  point P80 (0, -0.28)
  dimension "d0" = 14.984
  dimension "d1" = 1
  dimension "d4" = 0.05
  dimension "d5" = 15.05
  dimension "d6" = 0.05
  dimension "d7" = 0.1
  dimension "d8" = 0.1
  dimension "d9" = 0.1
  dimension "d10" = 0.1
  dimension "d13" = 0.2
  dimension "d19" = 0.23
  dimension "d20" = 15.05
  dimension "d21" = 0.23
  dimension "d22" = 0.05
  dimension "d23" = 0.15
  dimension "d24" = 0.1
  dimension "d25" = 0.1
  dimension "d26" = 0.1
  dimension "d34" = 0
  dimension "d36" = 0.05
  dimension "d37" = 0.1
  dimension "d40" = 0.2
  constraints: 1214 end point, 82 point on line, 9 perpendicular, 5 horizontal, 3 parallel, 3 vertical, 1 midpoint, 1387 other
  measures "d0" distance of L1.end L2.end
  measures "d1" distance of L0.end L1.end
  measures "d4" distance of L4.start L4.end
  measures "d5" distance of L6.start L6.end
  measures "d6" distance of L6.end L7.end
  measures "d7" distance of L7.end L8.end
  measures "d8" distance of L8.end L9.end
  measures "d9" distance of L9.end L10.end
  measures "d10" distance of L10.end L11.end
  measures "d13" distance of L7.end L12.start
  measures "d19" distance between parallel lines of L0 L6
  measures "d20" distance of L306.start L306.end
  measures "d21" distance between parallel lines of L2 L306
  measures "d22" distance of L306.start L307.end
  measures "d23" distance of L307.end L308.end
  measures "d24" distance of L308.end L309.end
  measures "d25" distance of L309.end L310.end
  measures "d26" distance of L310.end L311.end
  measures "d34" distance from line of point (0.205, -0.67) L303
  measures "d36" distance of L306.end L312.end
  measures "d37" distance of L311.end L313.end
  measures "d40" distance of L308.end L314.start
extrude "Extrusión1" add sketch "Boceto1" along normal blind 0.011 contours L6 L1 L8 L9 L10 L11 L12 L13 L14 L15 L16 L17 L18 L19 L20 L21 L22 L23 L24 L25 L26 L27 L28 L29 L30 L31 L32 L33 L34 L35 L36 L37 L38 L39 L40 L41 L42 L43 L44 L45 L46 L47 L48 L49 L50 L51 L52 L53 L54 L55 L56 L57 L58 L59 L60 L61 L62 L63 L64 L65 L66 L67 L68 L69 L70 L71 L72 L73 L74 L75 L76 L77 L78 L79 L80 L81 L82 L83 L84 L85 L86 L87 L88 L89 L90 L91 L92 L93 L94 L95 L96 L97 L98 L99 L100 L101 L102 L103 L104 L105 L106 L107 L108 L109 L110 L111 L112 L113 L114 L115 L116 L117 L118 L119 L120 L121 L122 L123 L124 L125 L126 L127 L128 L129 L130 L131 L132 L133 L134 L135 L136 L137 L138 L139 L140 L141 L142 L143 L144 L145 L146 L147 L148 L149 L150 L151 L152 L153 L154 L155 L156 L157 L158 L159 L160 L161 L162 L163 L164 L165 L166 L167 L168 L169 L170 L171 L172 L173 L174 L175 L176 L177 L178 L179 L180 L181 L182 L183 L184 L185 L186 L187 L188 L189 L190 L191 L192 L193 L194 L195 L196 L197 L198 L199 L200 L201 L202 L203 L204 L205 L206 L207 L208 L209 L210 L211 L212 L213 L214 L215 L216 L217 L218 L219 L220 L221 L222 L223 L224 L225 L226 L227 L228 L229 L230 L231 L232 L233 L234 L235 L236 L237 L238 L239 L240 L241 L242 L243 L244 L245 L246 L247 L248 L249 L250 L251 L252 L253 L254 L255 L256 L257 L258 L259 L260 L261 L262 L263 L264 L265 L266 L267 L268 L269 L270 L271 L272 L273 L274 L275 L276 L277 L278 L279 L280 L281 L282 L283 L284 L285 L286 L287 L288 L289 L290 L291 L292 L293 L294 L295 L296 L297 L298 L299 L300 L301 L302 L303 L304 L3 | L308 L309 L310 L311 L313 L314 L315 L316 L317 L318 L319 L320 L321 L322 L323 L324 L325 L326 L327 L328 L329 L330 L331 L332 L333 L334 L335 L336 L337 L338 L339 L340 L341 L342 L343 L344 L345 L346 L347 L348 L349 L350 L351 L352 L353 L354 L355 L356 L357 L358 L359 L360 L361 L362 L363 L364 L365 L366 L367 L368 L369 L370 L371 L372 L373 L374 L375 L376 L377 L378 L379 L380 L381 L382 L383 L384 L385 L386 L387 L388 L389 L390 L391 L392 L393 L394 L395 L396 L397 L398 L399 L400 L401 L402 L403 L404 L405 L406 L407 L408 L409 L410 L411 L412 L413 L414 L415 L416 L417 L418 L419 L420 L421 L422 L423 L424 L425 L426 L427 L428 L429 L430 L431 L432 L433 L434 L435 L436 L437 L438 L439 L440 L441 L442 L443 L444 L445 L446 L447 L448 L449 L450 L451 L452 L453 L454 L455 L456 L457 L458 L459 L460 L461 L462 L463 L464 L465 L466 L467 L468 L469 L470 L471 L472 L473 L474 L475 L476 L477 L478 L479 L480 L481 L482 L483 L484 L485 L486 L487 L488 L489 L490 L491 L492 L493 L494 L495 L496 L497 L498 L499 L500 L501 L502 L503 L504 L505 L506 L507 L508 L509 L510 L511 L512 L513 L514 L515 L516 L517 L518 L519 L520 L521 L522 L523 L524 L525 L526 L527 L528 L529 L530 L531 L532 L533 L534 L535 L536 L537 L538 L539 L540 L541 L542 L543 L544 L545 L546 L547 L548 L549 L550 L551 L552 L553 L554 L555 L556 L557 L558 L559 L560 L561 L562 L563 L564 L565 L566 L567 L568 L569 L570 L571 L572 L573 L574 L575 L576 L577 L578 L579 L580 L581 L582 L583 L584 L585 L586 L587 L588 L589 L590 L591 L592 L593 L594 L595 L596 L597 L598 L599 L600 L601 L602 L603 L604 L605 L606 L1 L306 L3
extrude "Extrusión3" add sketch "Boceto1" along normal blind 0.01 separate body contours L0 L1 L6 L3 | L304 L303 L302 L301 L300 L299 L298 L297 L296 L295 L294 L293 L292 L291 L290 L289 L288 L287 L286 L285 L284 L283 L282 L281 L280 L279 L278 L277 L276 L275 L274 L273 L272 L271 L270 L269 L268 L267 L266 L265 L264 L263 L262 L261 L260 L259 L258 L257 L256 L255 L254 L253 L252 L251 L250 L249 L248 L247 L246 L245 L244 L243 L242 L241 L240 L239 L238 L237 L236 L235 L234 L233 L232 L231 L230 L229 L228 L227 L226 L225 L224 L223 L222 L221 L220 L219 L218 L217 L216 L215 L214 L213 L212 L211 L210 L209 L208 L207 L206 L205 L204 L203 L202 L201 L200 L199 L198 L197 L196 L195 L194 L193 L192 L191 L190 L189 L188 L187 L186 L185 L184 L183 L182 L181 L180 L179 L178 L177 L176 L175 L174 L173 L172 L171 L170 L169 L168 L167 L166 L165 L164 L163 L162 L161 L160 L159 L158 L157 L156 L155 L154 L153 L152 L151 L150 L149 L148 L147 L146 L145 L144 L143 L142 L141 L140 L139 L138 L137 L136 L135 L134 L133 L132 L131 L130 L129 L128 L127 L126 L125 L124 L123 L122 L121 L120 L119 L118 L117 L116 L115 L114 L113 L112 L111 L110 L109 L108 L107 L106 L105 L104 L103 L102 L101 L100 L99 L98 L97 L96 L95 L94 L93 L92 L91 L90 L89 L88 L87 L86 L85 L84 L83 L82 L81 L80 L79 L78 L77 L76 L75 L74 L73 L72 L71 L70 L69 L68 L67 L66 L65 L64 L63 L62 L61 L60 L59 L58 L57 L56 L55 L54 L53 L52 L51 L50 L49 L48 L47 L46 L45 L44 L43 L42 L41 L40 L39 L38 L37 L36 L35 L34 L33 L32 L31 L30 L29 L28 L27 L26 L25 L24 L23 L22 L21 L20 L19 L18 L17 L16 L15 L14 L13 L12 L11 L10 L9 L8 L1 L606 L605 L604 L603 L602 L601 L600 L599 L598 L597 L596 L595 L594 L593 L592 L591 L590 L589 L588 L587 L586 L585 L584 L583 L582 L581 L580 L579 L578 L577 L576 L575 L574 L573 L572 L571 L570 L569 L568 L567 L566 L565 L564 L563 L562 L561 L560 L559 L558 L557 L556 L555 L554 L553 L552 L551 L550 L549 L548 L547 L546 L545 L544 L543 L542 L541 L540 L539 L538 L537 L536 L535 L534 L533 L532 L531 L530 L529 L528 L527 L526 L525 L524 L523 L522 L521 L520 L519 L518 L517 L516 L515 L514 L513 L512 L511 L510 L509 L508 L507 L506 L505 L504 L503 L502 L501 L500 L499 L498 L497 L496 L495 L494 L493 L492 L491 L490 L489 L488 L487 L486 L485 L484 L483 L482 L481 L480 L479 L478 L477 L476 L475 L474 L473 L472 L471 L470 L469 L468 L467 L466 L465 L464 L463 L462 L461 L460 L459 L458 L457 L456 L455 L454 L453 L452 L451 L450 L449 L448 L447 L446 L445 L444 L443 L442 L441 L440 L439 L438 L437 L436 L435 L434 L433 L432 L431 L430 L429 L428 L427 L426 L425 L424 L423 L422 L421 L420 L419 L418 L417 L416 L415 L414 L413 L412 L411 L410 L409 L408 L407 L406 L405 L404 L403 L402 L401 L400 L399 L398 L397 L396 L395 L394 L393 L392 L391 L390 L389 L388 L387 L386 L385 L384 L383 L382 L381 L380 L379 L378 L377 L376 L375 L374 L373 L372 L371 L370 L369 L368 L367 L366 L365 L364 L363 L362 L361 L360 L359 L358 L357 L356 L355 L354 L353 L352 L351 L350 L349 L348 L347 L346 L345 L344 L343 L342 L341 L340 L339 L338 L337 L336 L335 L334 L333 L332 L331 L330 L329 L328 L327 L326 L325 L324 L323 L322 L321 L320 L319 L318 L317 L316 L315 L314 L313 L311 L310 L309 L308 L3 | L306 L1 L2 L3
sketch "Boceto3" plane through (0, 0, 0) normal (1, 0, 0) x (0, 1, 0)
  point P0 (0, 0)
